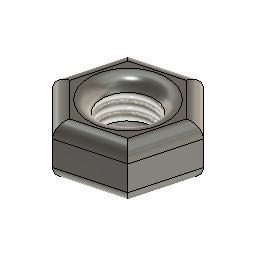
Nut-5 (Autodesk Fusion 360 design; units mm, degrees)
part number: 2026-04-30-21-03-03-585
Autodesk Fusion 360 part; units mm, degrees
sketch "Sketch1" plane through (0, 0, 0) normal (0, 0, 1) x (1, 0, 0)
  line L0 (3.5355, -3.5355) -> (4.8296, 1.2941)
  line L1 (4.8296, 1.2941) -> (1.2941, 4.8296)
  line L2 (1.2941, 4.8296) -> (-3.5355, 3.5355)
  line L3 (-3.5355, 3.5355) -> (-4.8296, -1.2941)
  line L4 (-4.8296, -1.2941) -> (-1.2941, -4.8296)
  line L5 (-1.2941, -4.8296) -> (3.5355, -3.5355)
  dimension "d1" = 5
  measures "d1" distance of L0.start origin
extrude "Extrude1" add sketch "Sketch1" along normal blind 4
sketch "Sketch2" plane through (0, 0, 4) normal (0, 0, 1) x (-1, 0, 0)
  line L0 (1.2941, 4.8296) -> (-3.5355, 3.5355)
  line L1 (-3.5355, 3.5355) -> (-4.8296, -1.2941)
  line L2 (-4.8296, -1.2941) -> (-1.2941, -4.8296)
  line L3 (-1.2941, -4.8296) -> (3.5355, -3.5355)
  line L4 (3.5355, -3.5355) -> (4.8296, 1.2941)
  line L5 (4.8296, 1.2941) -> (1.2941, 4.8296)
  circle A0 centre (0, 0) radius 2.5
  dimension "d4" = 5
  constraint coincident A0.centre origin
  measures "d4" diameter of A0
extrude "Extrude2" cut sketch "Sketch2" against normal blind 5 contours A0
fillet "Fillet1" radius 1 2 edges at (2.3308, -0.904, 4) (2.3308, 0.904, 0)
fillet "Fillet2" radius 1 12 edges at (-1.1207, 4.1826, 4) (-4.1826, 1.1207, 4) (3.0619, 3.0619, 4) (4.1826, -1.1207, 4) (1.1207, -4.1826, 4) (-3.0619, -3.0619, 4) (-4.1826, 1.1207, 0) (-1.1207, 4.1826, 0) (-3.0619, -3.0619, 0) (4.1826, -1.1207, 0) (3.0619, 3.0619, 0) (1.1207, -4.1826, 0)
thread "Thread1" "ISO Metric profile 5.0 M5x0.8 M5x0.8 6H" major diameter 5.12 minor diameter 4.234 pitch 0.8 angle 60 resizes the face on face at (-2.4876, 0.2489, 2.3333)
